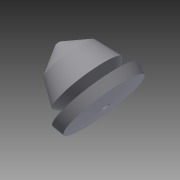
# Autodesk Inventor part: Part1
Saved by Autodesk Inventor 2015 (Build 190159000, 159)
## iProperties
Created: 2015-01-27
Part Number: Part1
Material: Generic
Document SubType Name: Modeling
Designer: PLTW-Stu-02
Density: 1 g/cm^3
Appearance: Default
Author: PLTW-Stu-02
Autodesk Inventor part; units mm, degrees
ref_plane "YZ Plane" through (0, 0, 0) normal (1, 0, 0) x (0, 1, 0)
ref_plane "XZ Plane" through (0, 0, 0) normal (0, 1, 0) x (-1, 0, 0)
ref_plane "XY Plane" through (0, 0, 0) normal (0, 0, 1) x (1, 0, 0)
sketch "Sketch1" plane through (0, 0, 0) normal (0, 0, 1) x (1, 0, 0)
  line L0 (13.0382, 19.2392) -> (29.1292, 26.2353)
  line L1 (29.1292, 26.2353) -> (45.6654, 22.7373)
  line L2 (45.6654, 22.7373) -> (48.273, 12.4976)
  line L3 (48.273, 12.4976) -> (54.5695, 23.1189)
  line L4 (54.5695, 23.1189) -> (59.8483, 17.6174)
  line L5 (59.8483, 17.6174) -> (48.273, -2.7666)
  line L6 (48.273, -2.7666) -> (13.0382, 19.2392)
  line L7 (11.0461, 18.3731) -> (46.9692, -5.0626) construction
  point P0 (0, 0)
  constraints: 16 end point, 1 point on line
revolve "Revolution1" add sketch "Sketch1" angle 360 about axis through (11.0461, 18.3731, 0) along (0.8375, -0.5464, 0)
body "Solid1"
